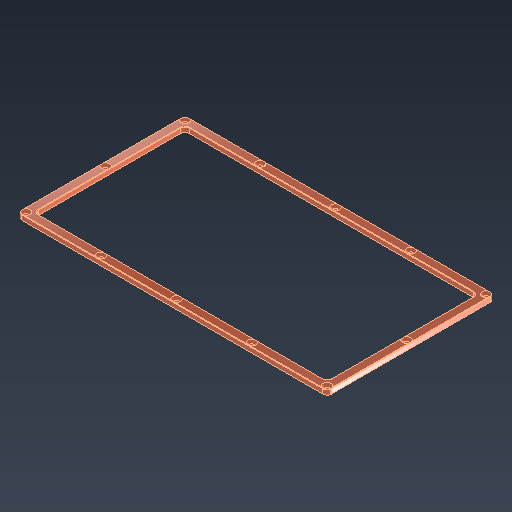
# Autodesk Inventor part: GRJ-04-106
Saved by Autodesk Inventor 2026.1 (Build 301233000, 233)
## iProperties
Company: Gree
Created: 2025-09-10
Part Number: GRJ-04-106
Material: Fenolite OR
Document SubType Name: Modeling
Designer: Willian Pinheiro
Density: 1.38 g/cm^3
Appearance: Suave - Laranja claro
Project: GRJ-04
Description: Suporte Estencil Auxiliar
Mass: 87.8839 g
Surface Area: 349.203 cm^2
Volume: 63.684 cm^3
Checked By: Antonio Lucas
Engr Approved By: Antonio Lucas
Mfg Approved By: Anderson Oliveira
Dimensões: 6 x 200 x 370 mm
Total: 1
Author: Willian Pinheiro
Title: Pasta Dissipador G
Revision Number: 00
Autodesk Inventor part; units mm, degrees
ref_plane "YZ Plane" through (0, 0, 0) normal (1, 0, 0) x (0, 1, 0)
ref_plane "XZ Plane" through (0, 0, 0) normal (0, 1, 0) x (-1, 0, 0)
ref_plane "XY Plane" through (0, 0, 0) normal (0, 0, 1) x (1, 0, 0)
sketch "Sketch1" plane through (0, 0, 0) normal (0, 0, 1) x (1, 0, 0)
  line L0 (-259, 0) -> (259, 0) construction
  line L1 (0, -140) -> (0, 140) construction
  line L2 (-185, 100) -> (185, 100)
  line L3 (185, 100) -> (185, -100)
  line L4 (185, -100) -> (-185, -100)
  line L5 (-185, -100) -> (-185, 100)
  line L6 (175, 90) -> (-175, 90)
  line L7 (-175, 90) -> (-175, -90)
  line L8 (-175, -90) -> (175, -90)
  line L9 (175, -90) -> (175, 90)
  line L10 (-180, 95) -> (180, 95) construction
  line L11 (180, 95) -> (180, -95) construction
  line L12 (180, -95) -> (-180, -95) construction
  line L13 (-180, -95) -> (-180, 95) construction
  point P0 (0, 0)
  point P1 (0, 95)
  point P2 (180, 0)
  point P3 (0, -95)
  point P4 (-180, 0)
  point P5 (-90, 95)
  point P6 (90, 95)
  point P7 (-90, -95)
  point P8 (90, -95)
  dimension "d0" = 370
  dimension "d1" = 200
  dimension "d2" = 10
  dimension "d3" = 5
  dimension "d19" = 90
  dimension "d20" = 90
  constraints: 24 end point, 6 parallel, 4 coincident, 4 midpoint, 3 perpendicular, 3 symmetric about line, 1 horizontal, 1 point on line, 8 other
  measures "d0" distance between parallel lines of L3 L5
  measures "d1" distance between parallel lines of L2 L4
  measures "d2" distance between parallel lines of L2 L6
  measures "d3" distance between parallel lines of L6 L10
  measures "d19" distance of point (0, 95) point (-90, 95)
  measures "d20" distance of point (-90, 95) point (-180, 95)
extrude "Extrusion1" add sketch "Sketch1" against normal blind 6 contours L2 L3 L4 L5 | L9 L8 L7 L6
extrude "Extrusion2" cut sketch "Sketch1" against normal blind 10 contours L9 L8 L7 L6
fillet "Fillet1" radius 5 8 edges at (-175, 90, -3) (-185, 100, -3) (185, 100, -3) (175, 90, -3) (185, -100, -3) (-185, -100, -3) (-175, -90, -3) (175, -90, -3)
chamfer "Chamfer1" distance 0.5 angle 45 16 edges at (0, 100, 0) (-183.5355, 98.5355, 0) (-185, 0, 0) (-183.5355, -98.5355, 0) (0, -100, 0) (183.5355, -98.5355, 0) (185, 0, 0) (183.5355, 98.5355, 0) (0, 90, 0) (173.5355, 88.5355, 0) (175, 0, 0) (173.5355, -88.5355, 0) (0, -90, 0) (-173.5355, -88.5355, 0) (-175, 0, 0) (-173.5355, 88.5355, 0)
hole "Hole1" at (-180, 95, 0) at (0, 95, 0) at (180, 95, 0) at (180, 0, 0) at (180, -95, 0) at (0, -95, 0) at (-180, 0, 0) at (-180, -95, 0) at (-90, 95, 0) at (90, 95, 0) at (90, -95, 0) at (-90, -95, 0) direction (0, 0, -1) diameter 4.5 end through all countersink diameter 10 countersink angle 90 clearance for "Countersunk Flat Head Hex Socket Screw ISO 10642" size "M4" standard "ISO"
equation "\"d19\" = d20"
body "Solid1"
